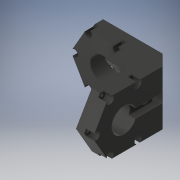
# Autodesk Inventor part: TARM03
Saved by Autodesk Inventor 2017 (Build 210142000, 142)
## iProperties
Created: 2018-10-19
Part Number: TARM03
Material: ABS Plastic
Document SubType Name: Modeling
Designer: Dell
Density: 1.06 g/cm^3
Appearance: Smooth - Black
Author: Dell
Autodesk Inventor part; units mm, degrees
ref_plane "YZ Plane" through (0, 0, 0) normal (1, 0, 0) x (0, 1, 0)
ref_plane "XZ Plane" through (0, 0, 0) normal (0, 1, 0) x (-1, 0, 0)
ref_plane "XY Plane" through (0, 0, 0) normal (0, 0, 1) x (1, 0, 0)
sketch "Sketch28" plane through (0, 0, 0) normal (0, 0, 1) x (1, 0, 0)
  line L0 (57.5, 0) -> (28.75, -49.7965)
  line L1 (28.75, -49.7965) -> (-28.75, -49.7965)
  line L2 (-28.75, -49.7965) -> (-57.5, 0)
  line L3 (-57.5, 0) -> (-28.75, 49.7965)
  line L4 (-28.75, 49.7965) -> (28.75, 49.7965)
  line L5 (28.75, 49.7965) -> (57.5, 0)
  circle A0 centre (51, 0) radius 2.5
  circle A1 centre (25.5, 44.1673) radius 2.5
  circle A2 centre (-25.5, 44.1673) radius 2.5
  circle A3 centre (-51, 0) radius 2.5
  circle A4 centre (-25.5, -44.1673) radius 2.5
  circle A5 centre (25.5, -44.1673) radius 2.5
  circle A6 centre (0, 0) radius 22.5
  line L6 (28.75, 49.7965) -> (100, 49.7965)
  line L7 (100, 49.7965) -> (100, -49.7965)
  line L8 (100, -49.7965) -> (28.75, -49.7965)
  dimension "d127" = 115
  dimension "d128" = 5
  dimension "d129" = 51
  dimension "d132" = 360
  dimension "d134" = 45
  dimension "d135" = 100
  constraints: 18 end point, 7 centre point, 2 coincident, 2 horizontal, 2 horizontal alignment, 1 perpendicular, 26 other
  measures "d127" distance of L0.start L2.end
  measures "d128" diameter of A0
  measures "d129" distance of A0.centre point (0, 0)
  measures "d134" diameter of A6
  measures "d135" distance from line of L7 point (0, 0)
extrude "Extrusion27" add sketch "Sketch28" along normal blind 30
sketch "Sketch29" plane through (100, -49.7965, 0) normal (1, 0, 0) x (0, 0, -1)
  line L0 (-33, 49.7965) -> (-61.75, 0)
  line L1 (-61.75, 0) -> (-119.25, 0)
  line L2 (-119.25, 0) -> (-148, 49.7965)
  line L3 (-148, 49.7965) -> (-119.25, 99.5929)
  line L4 (-119.25, 99.5929) -> (-61.75, 99.5929)
  line L5 (-61.75, 99.5929) -> (-33, 49.7965)
  line L6 (0, 0) -> (0, 99.5929) projected
  line L7 (-61.75, 99.5929) -> (0, 99.5929)
  line L8 (0, 96.4638) -> (-30, 96.4638) projected
  line L9 (0, 0) -> (-61.75, 0)
  circle A0 centre (-39.5, 49.7965) radius 2.5
  circle A1 centre (-65, 93.9638) radius 2.5
  circle A2 centre (-116, 93.9638) radius 2.5
  circle A3 centre (-141.5, 49.7965) radius 2.5
  circle A4 centre (-116, 5.6292) radius 2.5
  circle A5 centre (-65, 5.6292) radius 2.5
  circle A6 centre (-90.5, 49.7965) radius 22.5
  line L10 (-30, 0) -> (-30, 99.5929) projected
  point P0 (0, 49.7965)
  point P1 (0, 49.7965)
  dimension "d139" = 5
  dimension "d140" = 51
  dimension "d143" = 360
  dimension "d145" = 45
  dimension "d155" = 3
  constraints: 16 end point, 7 centre point, 4 horizontal alignment, 2 parallel, 1 coincident, 1 midpoint, 26 other
  measures "d139" diameter of A0
  measures "d140" distance of A0.centre point (-90.5, 49.796)
  measures "d145" diameter of A6
  measures "d155" distance from line of L10 L0.start
extrude "Extrusion28" add sketch "Sketch29" against normal blind 30
sketch "Sketch30" plane through (-28.75, 49.7965, 0) normal (0, 1, 0) x (1, 0, 0)
  line L0 (98.75, -30) -> (0, -30) projected
  line L1 (63.75, -30) -> (98.75, -90)
  line L2 (98.75, -30) -> (98.75, -119.25) projected
  line L3 (98.75, -30) -> (98.75, -90)
  line L4 (98.75, -30) -> (63.75, -30)
  line L5 (63.75, -30) -> (63.75, -90)
  line L6 (63.75, -90) -> (98.75, -90)
  point P0 (28.75, 0)
  dimension "d148" = 35
  dimension "d149" = 60
  constraints: 10 end point, 2 perpendicular, 2 point on line, 1 collinear, 1 vertical
  measures "d148" distance of L0.start L1.start
  measures "d149" distance of L0.start L1.end
extrude "Extrusion29" add sketch "Sketch30" against normal blind 99.5929
sketch "Sketch31" plane through (70, -49.7965, 0) normal (-1, 0, 0) x (0, 0, 1)
  arc A0 (90, 27.302) -> (90, 72.2909) centre (90.5, 49.7965) ccw projected
  line L0 (149, 49.7965) -> (119.75, -0.866)
  line L1 (119.75, -0.866) -> (61.25, -0.866)
  line L2 (61.25, -0.866) -> (32, 49.7965)
  line L3 (32, 49.7965) -> (61.25, 100.4589)
  line L4 (61.25, 100.4589) -> (119.75, 100.4589)
  line L5 (119.75, 100.4589) -> (149, 49.7965)
  point P0 (0, 49.7965)
  dimension "d152" = 117
  constraints: 12 end point, 1 coincident, 1 horizontal alignment, 13 other
  measures "d152" distance of L0.start L2.end
extrude "Extrusion30" cut sketch "Sketch31" along normal through all
sketch "Sketch32" plane through (70, -49.7965, 0) normal (-1, 0, 0) x (0, 0, 1)
  line L0 (103.5, 0) -> (76.5, 0)
  line L1 (76.5, 0) -> (76.5, -4)
  line L2 (76.5, -4) -> (103.5, -4)
  line L3 (103.5, -4) -> (103.5, 0)
  line L4 (60.75, 0) -> (119.25, 0) construction
  circle A0 centre (90.5, 49.7965) radius 22.5 construction
  line L5 (140.125, 36.1566) -> (126.625, 12.7739)
  line L6 (126.625, 12.7739) -> (130.0891, 10.7739)
  line L7 (130.0891, 10.7739) -> (143.5891, 34.1566)
  line L8 (143.5891, 34.1566) -> (140.125, 36.1566)
  line L9 (127.125, 85.953) -> (140.625, 62.5703)
  line L10 (140.625, 62.5703) -> (144.0891, 64.5703)
  line L11 (144.0891, 64.5703) -> (130.5891, 87.953)
  line L12 (130.5891, 87.953) -> (127.125, 85.953)
  line L13 (77.5, 99.5929) -> (104.5, 99.5929)
  line L14 (104.5, 99.5929) -> (104.5, 103.5929)
  line L15 (104.5, 103.5929) -> (77.5, 103.5929)
  line L16 (77.5, 103.5929) -> (77.5, 99.5929)
  line L17 (40.875, 63.4364) -> (54.375, 86.819)
  line L18 (54.375, 86.819) -> (50.9109, 88.819)
  line L19 (50.9109, 88.819) -> (37.4109, 65.4364)
  line L20 (37.4109, 65.4364) -> (40.875, 63.4364)
  line L21 (53.875, 13.6399) -> (40.375, 37.0226)
  line L22 (40.375, 37.0226) -> (36.9109, 35.0226)
  line L23 (36.9109, 35.0226) -> (50.4109, 11.6399)
  line L24 (50.4109, 11.6399) -> (53.875, 13.6399)
  point P0 (0, 49.7965)
  point P1 (90, 0)
  point P2 (133.375, 24.4652)
  point P3 (133.875, 74.2617)
  point P4 (91, 99.5929)
  point P5 (47.625, 75.1277)
  point P6 (47.125, 25.3312)
  dimension "d156" = 27
  dimension "d157" = 4
  dimension "d160" = 360
  constraints: 48 end point, 2 midpoint, 2 parallel, 1 horizontal, 1 perpendicular, 55 other
  measures "d156" distance of L1.end L2.end
  measures "d157" distance of L2.end L0.start
extrude "Extrusion31" cut sketch "Sketch32" along normal through all
sketch "Sketch37" plane through (100, -49.7965, 0) normal (1, 0, 0) x (0, 0, -1)
  line L0 (-27, 41.2965) -> (-15, 41.2965)
  line L1 (-15, 41.2965) -> (-15, 58.2965)
  line L2 (-15, 58.2965) -> (-27, 58.2965)
  line L3 (-27, 58.2965) -> (-27, 41.2965)
  line L4 (0, 0) -> (0, 99.5929) projected
  point P0 (0, 49.7965)
  point P1 (-15, 49.7965)
  point P2 (0, 49.7965)
  dimension "d182" = 12
  dimension "d183" = 17
  dimension "d184" = 15
  constraints: 8 end point, 2 midpoint, 2 parallel, 1 horizontal, 1 horizontal alignment, 1 perpendicular
  measures "d182" distance of L2.end L1.end
  measures "d183" distance of L1.end L0.end
  measures "d184" distance between parallel lines of L4 L1
extrude "Extrusion36" cut sketch "Sketch37" against normal blind 100
sketch "Sketch38" plane through (100, -49.7965, 0) normal (1, 0, 0) x (0, 0, -1)
  line L0 (-15, 58.2965) -> (-15, 41.2965) projected
  line L1 (-27, 58.2965) -> (-15, 58.2965) projected
  line L2 (-27, 41.2965) -> (-27, 58.2965) projected
  line L3 (-15, 41.2965) -> (-27, 41.2965) projected
  line L4 (-15, 41.2965) -> (-100, 41.2965)
  line L5 (-100, 41.2965) -> (-100, 58.2965)
  line L6 (-100, 58.2965) -> (-15, 58.2965)
  line L7 (-15, 58.2965) -> (-15, 41.2965)
  point P0 (0, 49.7965)
  dimension "d187" = 85
  constraints: 8 end point, 2 parallel, 1 horizontal, 1 perpendicular
  measures "d187" distance of L5.end L0.start
extrude "Extrusion37" cut sketch "Sketch38" against normal blind 12 contours L2 L4 L5 L6
sketch "Sketch39" plane through (0, 0, 30) normal (0, 0, 1) x (1, 0, 0)
  circle A0 centre (-51, 0) radius 2.5 projected
  circle A1 centre (-51, 0) radius 6.5
  circle A2 centre (-25.5, -44.1673) radius 6.5
  circle A3 centre (25.5, -44.1673) radius 6.5
  circle A4 centre (51, 0) radius 6.5
  circle A5 centre (25.5, 44.1673) radius 6.5
  circle A6 centre (-25.5, 44.1673) radius 6.5
  point P0 (0, 0)
  dimension "d190" = 13
  dimension "d193" = 360
  constraints: 6 centre point, 1 coincident, 13 other
  measures "d190" diameter of A1
extrude "Extrusion38" cut sketch "Sketch39" along normal blind 15 and the other way blind 15 contours A0 | A1 | A2 | A3 | A4 | A5 | A6
sketch "Sketch40" plane through (100, -49.7965, 0) normal (1, 0, 0) x (0, 0, -1)
  circle A0 centre (-141.5, 49.7965) radius 2.5 projected
  circle A1 centre (-141.5, 49.7965) radius 6.5
  arc A2 (-69.6673, 58.2965) -> (-69.6673, 41.2965) centre (-90.5, 49.7965) ccw projected
  circle A3 centre (-116, 5.6292) radius 6.5
  circle A4 centre (-65, 5.6292) radius 6.5
  circle A5 centre (-39.5, 49.7965) radius 6.5
  circle A6 centre (-65, 93.9638) radius 6.5
  circle A7 centre (-116, 93.9638) radius 6.5
  point P0 (0, 49.7965)
  dimension "d199" = 13
  dimension "d202" = 360
  constraints: 6 centre point, 1 coincident, 13 other
  measures "d199" diameter of A1
extrude "Extrusion39" cut sketch "Sketch40" along normal blind 15 and the other way blind 15 contours A0 | A1 | A3 | A4 | A5 | A6 | A7
chamfer "Chamfer2" distance 20 angle 45 1 edges at (100, 0, 0)
body "Solid2"
